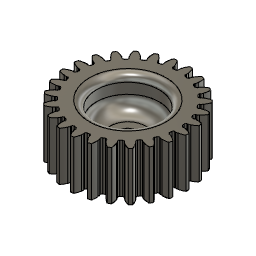
_motor gear.89c0d897-75a3-4985-b3bd-b82dc4103b69 (Autodesk Fusion 360 design; units mm, degrees)
description: Spur Gear; Module: 1.270000; Num Teeth: 25; Pressure Angle: 20.000000;
Autodesk Fusion 360 part; units mm, degrees
sketch "Sketch1" plane through (0, 0, 0) normal (0, 1, 0) x (1, 0, 0) in component "Spur Gear (25 teeth)"
  circle A0 centre (0, 0) radius 15.875 construction
sketch "sketch 16717" plane through (0, 0, 0) normal (0, 1, 0) x (1, 0, 0)
  arc A0 (14.1346, -2.0844) -> (14.4612, -2.5368) centre (14.5304, -2.1428) ccw
  spline S0 degree 3 poles (16.7153, -3.8203) (16.1288, -3.2859) (15.6262, -2.9744) (15.269, -2.7969) knots 0 0 0 0 1 1 1 1
  circle A1 centre (0, 0) radius 2.5
  line L0 (14.7175, -2.5817) -> (14.4612, -2.5368)
  arc A2 (14.1346, -2.0844) -> (14.2089, -1.4962) centre (0, 0) ccw
  spline S1 degree 3 poles (12.0329, -9.8069) (11.842, -9.5326) (11.7016, -9.3961) (11.6533, -9.3526) knots 0 0 0 0 1 1 1 1
  arc A3 (11.3821, -8.636) -> (11.4504, -9.1897) centre (11.7008, -8.8778) ccw
  arc A4 (11.3821, -8.636) -> (11.7306, -8.1563) centre (0, 0) ccw
  arc A5 (12.2783, -8.0502) -> (11.7306, -8.1563) centre (12.059, -8.3847) ccw
  arc A6 (14.8001, -8.6575) -> (15.2401, -7.8572) centre (0, 0) ccw
  spline S2 degree 3 poles (13.0445, -8.4135) (13.4271, -8.5286) (14.0067, -8.6456) (14.8001, -8.6575) knots 0 0 0 0 1 1 1 1
  spline S3 degree 3 poles (12.8073, -11.4004) (12.5507, -10.6496) (12.2604, -10.1345) (12.0329, -9.8069) knots 0 0 0 0 1 1 1 1
  spline S4 degree 3 poles (15.269, -2.7969) (14.9696, -2.6485) (14.7808, -2.5966) (14.7175, -2.5817) knots 0 0 0 0 1 1 1 1
  line L1 (11.6533, -9.3526) -> (11.4504, -9.1897)
  arc A7 (13.1722, -5.5341) -> (13.3761, -6.0534) centre (13.541, -5.689) ccw
  arc A8 (13.8946, -4.7438) -> (13.3904, -4.9828) centre (13.7653, -5.1223) ccw
  arc A9 (-4.1322, 13.6769) -> (-4.6961, 13.4937) centre (0, 0) ccw
  spline S5 degree 3 poles (-3.9705, 15.0067) (-3.9773, 14.6726) (-3.9439, 14.4796) (-3.9304, 14.416) knots 0 0 0 0 1 1 1 1
  arc A10 (-4.1322, 13.6769) -> (-3.862, 14.165) centre (-4.2479, 14.0598) ccw
  spline S6 degree 3 poles (14.727, -4.9052) (15.1263, -4.9214) (15.7167, -4.8906) (16.4882, -4.7049) knots 0 0 0 0 1 1 1 1
  line L2 (13.6131, -6.1607) -> (13.3761, -6.0534)
  spline S7 degree 3 poles (15.2401, -7.8572) (14.8049, -7.1938) (14.3955, -6.7671) (14.0937, -6.5063) knots 0 0 0 0 1 1 1 1
  spline S8 degree 3 poles (14.0937, -6.5063) (13.8406, -6.2881) (13.6707, -6.1908) (13.6131, -6.1607) knots 0 0 0 0 1 1 1 1
  arc A11 (13.1722, -5.5341) -> (13.3904, -4.9828) centre (0, 0) ccw
  spline S9 degree 3 poles (14.1408, -4.8278) (14.2034, -4.8453) (14.3939, -4.8907) (14.727, -4.9052) knots 0 0 0 0 1 1 1 1
  line L3 (12.2783, -8.0502) -> (12.4959, -8.1928)
  spline S10 degree 3 poles (12.4959, -8.1928) (12.5522, -8.2253) (12.7254, -8.3167) (13.0445, -8.4135) knots 0 0 0 0 1 1 1 1
  spline S11 degree 3 poles (-1.6525, 14.8505) (-1.6634, 14.9146) (-1.7034, 15.1064) (-1.8321, 15.4139) knots 0 0 0 0 1 1 1 1
  spline S12 degree 3 poles (-1.8321, 15.4139) (-1.9874, 15.7821) (-2.2667, 16.3033) (-2.7632, 16.9222) knots 0 0 0 0 1 1 1 1
  line L4 (13.8946, -4.7438) -> (14.1408, -4.8278)
  arc A12 (16.4882, -4.7049) -> (16.7153, -3.8203) centre (0, 0) ccw
  arc A13 (-2.7632, 16.9222) -> (-3.6603, 16.7511) centre (0, 0) ccw
  spline S13 degree 3 poles (-3.6603, 16.7511) (-3.8941, 15.9928) (-3.9619, 15.4055) (-3.9705, 15.0067) knots 0 0 0 0 1 1 1 1
  spline S14 degree 3 poles (-5.6078, 14.474) (-5.8498, 14.792) (-6.25, 15.2273) (-6.8848, 15.7034) knots 0 0 0 0 1 1 1 1
  spline S15 degree 3 poles (-7.5778, 13.5478) (-7.5012, 13.2225) (-7.4209, 13.0439) (-7.392, 12.9856) knots 0 0 0 0 1 1 1 1
  spline S16 degree 3 poles (-7.7111, 15.3145) (-7.749, 14.522) (-7.6687, 13.9362) (-7.5778, 13.5478) knots 0 0 0 0 1 1 1 1
  spline S17 degree 3 poles (-8.6024, 12.2175) (-8.6428, 12.2685) (-8.7702, 12.4172) (-9.0312, 12.6247) knots 0 0 0 0 1 1 1 1
  arc A14 (-7.4037, 12.2196) -> (-7.2633, 12.7596) centre (-7.611, 12.5617) ccw
  arc A15 (-7.4037, 12.2196) -> (-7.9043, 11.9019) centre (0, 0) ccw
  spline S18 degree 3 poles (-10.7089, 11.2377) (-10.5539, 10.9416) (-10.4317, 10.7886) (-10.3892, 10.7394) knots 0 0 0 0 1 1 1 1
  line L5 (-10.3892, 10.7394) -> (-10.2083, 10.5524)
  spline S19 degree 3 poles (-11.2774, 12.9157) (-11.117, 12.1386) (-10.8935, 11.5912) (-10.7089, 11.2377) knots 0 0 0 0 1 1 1 1
  spline S20 degree 3 poles (-9.0312, 12.6247) (-9.3447, 12.8725) (-9.8405, 13.1947) (-10.5738, 13.4978) knots 0 0 0 0 1 1 1 1
  arc A16 (-10.5738, 13.4978) -> (-11.2774, 12.9157) centre (0, 0) ccw
  arc A17 (-5.2016, 13.7298) -> (-4.6961, 13.4937) centre (-4.8275, 13.8715) ccw
  arc A18 (-6.8848, 15.7034) -> (-7.7111, 15.3145) centre (0, 0) ccw
  line L6 (-5.2016, 13.7298) -> (-5.2938, 13.973)
  line L7 (-7.392, 12.9856) -> (-7.2633, 12.7596)
  line L8 (-3.9304, 14.416) -> (-3.862, 14.165)
  arc A19 (-8.4526, 12.0048) -> (-7.9043, 11.9019) centre (-8.1256, 12.2351) ccw
  line L9 (-8.4526, 12.0048) -> (-8.6024, 12.2175)
  spline S21 degree 3 poles (-5.2938, 13.973) (-5.3202, 14.0324) (-5.4067, 14.2082) (-5.6078, 14.474) knots 0 0 0 0 1 1 1 1
  arc A20 (-12.3747, 7.1413) -> (-12.5119, 7.6822) centre (-12.7212, 7.3413) ccw
  spline S22 degree 3 poles (-13.9961, 6.7123) (-14.3902, 6.7785) (-14.9799, 6.8219) (-15.7685, 6.7343) knots 0 0 0 0 1 1 1 1
  spline S23 degree 3 poles (-11.3705, 9.6944) (-11.4223, 9.7337) (-11.5827, 9.846) (-11.8871, 9.9821) knots 0 0 0 0 1 1 1 1
  arc A21 (-10.21, 9.9945) -> (-10.6158, 9.5623) centre (0, 0) ccw
  spline S24 degree 3 poles (-17.0623, 1.6952) (-16.4134, 1.2386) (-15.8758, 0.9925) (-15.4992, 0.8612) knots 0 0 0 0 1 1 1 1
  arc A22 (-14.2844, 0.2964) -> (-14.2844, -0.2964) centre (0, 0) ccw
  spline S25 degree 3 poles (-13.1672, 8.2214) (-12.9434, 7.9732) (-12.7869, 7.8554) (-12.7336, 7.8183) knots 0 0 0 0 1 1 1 1
  line L10 (-14.925, 0.7168) -> (-14.6652, 0.7043)
  spline S26 degree 3 poles (-14.7981, 4.6886) (-14.5196, 4.5038) (-14.3388, 4.4286) (-14.2778, 4.4059) knots 0 0 0 0 1 1 1 1
  arc A23 (-11.1725, 9.5256) -> (-10.6158, 9.5623) centre (-10.913, 9.83) ccw
  spline S27 degree 3 poles (-16.1047, 5.8852) (-15.5897, 5.2815) (-15.1302, 4.9095) (-14.7981, 4.6886) knots 0 0 0 0 1 1 1 1
  spline S28 degree 3 poles (-15.2257, 3.0207) (-15.6238, 2.9868) (-16.2058, 2.8822) (-16.9478, 2.6013) knots 0 0 0 0 1 1 1 1
  spline S29 degree 3 poles (-15.4992, 0.8612) (-15.1835, 0.7515) (-14.9897, 0.7236) (-14.925, 0.7168) knots 0 0 0 0 1 1 1 1
  spline S30 degree 3 poles (-15.4985, -0.8607) (-15.8758, -0.9925) (-16.4134, -1.2386) (-17.0623, -1.6952) knots 0 0 0 0 1 1 1 1
  arc A24 (-13.5983, 10.4442) -> (-14.1351, 9.7054) centre (0, 0) ccw
  line L11 (-12.7336, 7.8183) -> (-12.5119, 7.6822)
  arc A25 (-17.0623, -1.6952) -> (-16.9478, -2.6013) centre (0, 0) ccw
  line L12 (-14.0293, -4.3292) -> (-14.2778, -4.4059)
  arc A26 (-16.9478, 2.6013) -> (-17.0623, 1.6952) centre (0, 0) ccw
  arc A27 (-13.9094, -3.2653) -> (-14.3796, -2.9649) centre (-14.2988, -3.3567) ccw
  spline S31 degree 3 poles (-11.8871, 9.9821) (-12.2524, 10.1442) (-12.8127, 10.3329) (-13.5983, 10.4442) knots 0 0 0 0 1 1 1 1
  line L13 (-14.2778, 4.4059) -> (-14.0293, 4.3292)
  spline S32 degree 3 poles (-16.9478, -2.6013) (-16.2058, -2.8822) (-15.6238, -2.9868) (-15.2264, -3.0204) knots 0 0 0 0 1 1 1 1
  line L14 (-14.6343, -3.0175) -> (-14.3796, -2.9649)
  arc A28 (-13.9094, -3.2653) -> (-13.7619, -3.8395) centre (0, 0) ccw
  spline S33 degree 3 poles (-14.6343, 3.0175) (-14.6987, 3.0269) (-14.8934, 3.0481) (-15.2257, 3.0207) knots 0 0 0 0 1 1 1 1
  spline S34 degree 3 poles (-15.2264, -3.0204) (-14.8934, -3.0481) (-14.6987, -3.0269) (-14.6343, -3.0175) knots 0 0 0 0 1 1 1 1
  arc A29 (-12.3747, 7.1413) -> (-12.6603, 6.6218) centre (0, 0) ccw
  line L15 (-11.1725, 9.5256) -> (-11.3705, 9.6944)
  arc A30 (-15.7685, 6.7343) -> (-16.1047, 5.8852) centre (0, 0) ccw
  spline S35 degree 3 poles (-13.4242, 6.5621) (-13.4841, 6.5872) (-13.6674, 6.6562) (-13.9961, 6.7123) knots 0 0 0 0 1 1 1 1
  line L16 (-13.1905, 6.4478) -> (-13.4242, 6.5621)
  arc A31 (-13.1905, 6.4478) -> (-12.6603, 6.6218) centre (-13.0148, 6.8072) ccw
  line L17 (-14.3796, 2.9649) -> (-14.6343, 3.0175)
  spline S36 degree 3 poles (-14.925, -0.7168) (-14.9897, -0.7236) (-15.1835, -0.7515) (-15.4985, -0.8607) knots 0 0 0 0 1 1 1 1
  arc A32 (-14.2844, 0.2964) -> (-14.6652, 0.7043) centre (-14.6843, 0.3047) ccw
  spline S37 degree 3 poles (-14.1351, 9.7054) (-13.7865, 8.9926) (-13.4339, 8.518) (-13.1672, 8.2214) knots 0 0 0 0 1 1 1 1
  line L18 (-14.6652, -0.7043) -> (-14.925, -0.7168)
  arc A33 (-13.7619, 3.8395) -> (-13.9094, 3.2653) centre (0, 0) ccw
  arc A34 (-14.3796, 2.9649) -> (-13.9094, 3.2653) centre (-14.2988, 3.3567) ccw
  arc A35 (-10.21, 9.9945) -> (-10.2083, 10.5524) centre (-10.4958, 10.2743) ccw
  arc A36 (-13.7619, 3.8395) -> (-14.0293, 4.3292) centre (-14.1472, 3.947) ccw
  arc A37 (-14.6652, -0.7043) -> (-14.2844, -0.2964) centre (-14.6843, -0.3047) ccw
  arc A38 (-4.6961, -13.4937) -> (-4.1322, -13.6769) centre (0, 0) ccw
  spline S38 degree 3 poles (2.0584, -15.386) (2.1069, -15.0554) (2.098, -14.8597) (2.0926, -14.7949) knots 0 0 0 0 1 1 1 1
  arc A39 (-12.6603, -6.6218) -> (-13.1905, -6.4478) centre (-13.0148, -6.8072) ccw
  arc A40 (3.4398, -14.2734) -> (2.9678, -13.9759) centre (3.0509, -14.3671) ccw
  arc A41 (-14.0293, -4.3292) -> (-13.7619, -3.8395) centre (-14.1472, -3.947) ccw
  arc A42 (-10.6158, -9.5623) -> (-11.1725, -9.5256) centre (-10.913, -9.83) ccw
  line L19 (-12.5119, -7.6822) -> (-12.7336, -7.8183)
  spline S39 degree 3 poles (-7.5778, -13.547) (-7.6687, -13.9362) (-7.749, -14.522) (-7.7111, -15.3145) knots 0 0 0 0 1 1 1 1
  arc A43 (-12.5119, -7.6822) -> (-12.3747, -7.1413) centre (-12.7212, -7.3413) ccw
  arc A44 (-0.2179, -14.6804) -> (-0.6011, -14.2749) centre (-0.6179, -14.6745) ccw
  arc A45 (-11.2774, -12.9157) -> (-10.5738, -13.4978) centre (0, 0) ccw
  line L20 (-5.2938, -13.973) -> (-5.2016, -13.7298)
  spline S40 degree 3 poles (-3.9708, -15.0059) (-3.9619, -15.4055) (-3.8941, -15.9928) (-3.6603, -16.7511) knots 0 0 0 0 1 1 1 1
  spline S41 degree 3 poles (-13.5983, -10.4442) (-12.8127, -10.3329) (-12.2524, -10.1442) (-11.8879, -9.9822) knots 0 0 0 0 1 1 1 1
  line L21 (-0.2179, -14.6804) -> (-0.2218, -14.9405)
  spline S42 degree 3 poles (-11.8879, -9.9822) (-11.5827, -9.846) (-11.4223, -9.7337) (-11.3705, -9.6944) knots 0 0 0 0 1 1 1 1
  spline S43 degree 3 poles (-0.1142, -15.522) (-0.0063, -15.9068) (0.2055, -16.4588) (0.6205, -17.1351) knots 0 0 0 0 1 1 1 1
  arc A46 (-12.6603, -6.6218) -> (-12.3747, -7.1413) centre (0, 0) ccw
  arc A47 (0.6205, -17.1351) -> (1.532, -17.0777) centre (0, 0) ccw
  arc A48 (-14.1351, -9.7054) -> (-13.5983, -10.4442) centre (0, 0) ccw
  arc A49 (-7.2633, -12.7596) -> (-7.4037, -12.2196) centre (-7.611, -12.5617) ccw
  arc A50 (-7.7111, -15.3145) -> (-6.8848, -15.7034) centre (0, 0) ccw
  spline S44 degree 3 poles (-6.8848, -15.7034) (-6.25, -15.2273) (-5.8498, -14.792) (-5.6085, -14.4745) knots 0 0 0 0 1 1 1 1
  spline S45 degree 3 poles (-15.7685, -6.7343) (-14.9799, -6.8219) (-14.3902, -6.7785) (-13.9969, -6.7121) knots 0 0 0 0 1 1 1 1
  arc A51 (-4.6961, -13.4937) -> (-5.2016, -13.7298) centre (-4.8275, -13.8715) ccw
  line L22 (-10.2083, -10.5524) -> (-10.3892, -10.7394)
  arc A52 (-16.1047, -5.8852) -> (-15.7685, -6.7343) centre (0, 0) ccw
  line L23 (-13.4242, -6.5621) -> (-13.1905, -6.4478)
  arc A53 (-1.1928, -14.2376) -> (-1.6237, -14.592) centre (-1.2262, -14.6362) ccw
  arc A54 (-10.2083, -10.5524) -> (-10.21, -9.9945) centre (-10.4958, -10.2743) ccw
  arc A55 (-10.6158, -9.5623) -> (-10.21, -9.9945) centre (0, 0) ccw
  spline S46 degree 3 poles (-14.7976, -4.688) (-15.1302, -4.9095) (-15.5897, -5.2815) (-16.1047, -5.8852) knots 0 0 0 0 1 1 1 1
  line L24 (-11.3705, -9.6944) -> (-11.1725, -9.5256)
  spline S47 degree 3 poles (-10.5738, -13.4978) (-9.8405, -13.1947) (-9.3447, -12.8725) (-9.032, -12.6249) knots 0 0 0 0 1 1 1 1
  line L25 (-7.2633, -12.7596) -> (-7.392, -12.9856)
  spline S48 degree 3 poles (-1.8327, -15.4145) (-1.7034, -15.1064) (-1.6634, -14.9146) (-1.6525, -14.8505) knots 0 0 0 0 1 1 1 1
  arc A56 (-1.1928, -14.2376) -> (-0.6011, -14.2749) centre (0, 0) ccw
  spline S49 degree 3 poles (-14.2778, -4.4059) (-14.3388, -4.4286) (-14.5196, -4.5038) (-14.7976, -4.688) knots 0 0 0 0 1 1 1 1
  line L26 (3.4398, -14.2734) -> (3.5007, -14.5263)
  arc A57 (-3.862, -14.165) -> (-4.1322, -13.6769) centre (-4.2479, -14.0598) ccw
  spline S50 degree 3 poles (-13.1668, -8.2207) (-13.4339, -8.518) (-13.7865, -8.9926) (-14.1351, -9.7054) knots 0 0 0 0 1 1 1 1
  arc A58 (-3.6603, -16.7511) -> (-2.7632, -16.9222) centre (0, 0) ccw
  spline S51 degree 3 poles (-3.9304, -14.416) (-3.9439, -14.4796) (-3.9773, -14.6726) (-3.9708, -15.0059) knots 0 0 0 0 1 1 1 1
  line L27 (-1.6525, -14.8505) -> (-1.6237, -14.592)
  arc A59 (-7.9043, -11.9019) -> (-8.4526, -12.0048) centre (-8.1256, -12.2351) ccw
  spline S52 degree 3 poles (-10.3892, -10.7394) (-10.4317, -10.7886) (-10.5539, -10.9416) (-10.7088, -11.2369) knots 0 0 0 0 1 1 1 1
  spline S53 degree 3 poles (-12.7336, -7.8183) (-12.7869, -7.8554) (-12.9434, -7.9732) (-13.1668, -8.2207) knots 0 0 0 0 1 1 1 1
  arc A60 (-7.9043, -11.9019) -> (-7.4037, -12.2196) centre (0, 0) ccw
  spline S54 degree 3 poles (-10.7088, -11.2369) (-10.8935, -11.5912) (-11.117, -12.1386) (-11.2774, -12.9157) knots 0 0 0 0 1 1 1 1
  line L28 (-3.862, -14.165) -> (-3.9304, -14.416)
  arc A61 (2.3854, -14.087) -> (2.9678, -13.9759) centre (0, 0) ccw
  line L29 (-8.6024, -12.2175) -> (-8.4526, -12.0048)
  spline S55 degree 3 poles (-0.2218, -14.9405) (-0.2191, -15.0055) (-0.2034, -15.2007) (-0.1142, -15.522) knots 0 0 0 0 1 1 1 1
  line L30 (2.0926, -14.7949) -> (2.0562, -14.5374)
  spline S56 degree 3 poles (1.532, -17.0777) (1.859, -16.3548) (1.9999, -15.7805) (2.0584, -15.386) knots 0 0 0 0 1 1 1 1
  arc A62 (4.8623, -16.4424) -> (5.7309, -16.1602) centre (0, 0) ccw
  spline S57 degree 3 poles (3.7496, -15.0627) (3.9498, -15.4086) (4.2922, -15.8906) (4.8623, -16.4424) knots 0 0 0 0 1 1 1 1
  spline S58 degree 3 poles (-13.9969, -6.7121) (-13.6674, -6.6562) (-13.4841, -6.5872) (-13.4242, -6.5621) knots 0 0 0 0 1 1 1 1
  spline S59 degree 3 poles (-7.392, -12.9856) (-7.4209, -13.0439) (-7.5012, -13.2225) (-7.5778, -13.547) knots 0 0 0 0 1 1 1 1
  spline S60 degree 3 poles (-2.7632, -16.9222) (-2.2667, -16.3033) (-1.9874, -15.7821) (-1.8327, -15.4145) knots 0 0 0 0 1 1 1 1
  arc A63 (2.3854, -14.087) -> (2.0562, -14.5374) centre (2.4522, -14.4813) ccw
  spline S61 degree 3 poles (-5.6085, -14.4745) (-5.4067, -14.2082) (-5.3202, -14.0324) (-5.2938, -13.973) knots 0 0 0 0 1 1 1 1
  spline S62 degree 3 poles (-9.032, -12.6249) (-8.7702, -12.4172) (-8.6428, -12.2685) (-8.6024, -12.2175) knots 0 0 0 0 1 1 1 1
  arc A64 (5.8138, -13.0512) -> (6.3502, -12.7987) centre (0, 0) ccw
  spline S63 degree 3 poles (5.7309, -16.1602) (5.8678, -15.3786) (5.8615, -14.7874) (5.82, -14.3907) knots 0 0 0 0 1 1 1 1
  line L31 (11.4504, 9.1897) -> (11.6533, 9.3526)
  arc A65 (11.7306, 8.1563) -> (12.2783, 8.0502) centre (12.059, 8.3847) ccw
  arc A66 (6.8814, -12.9696) -> (6.3502, -12.7987) centre (6.528, -13.157) ccw
  arc A67 (11.7306, 8.1563) -> (11.3821, 8.636) centre (0, 0) ccw
  spline S64 degree 3 poles (15.4842, -1.0886) (15.875, -1.0051) (16.4392, -0.8284) (17.1402, -0.4566) knots 0 0 0 0 1 1 1 1
  line L32 (13.3761, 6.0534) -> (13.6131, 6.1607)
  arc A68 (13.3904, 4.9828) -> (13.8946, 4.7438) centre (13.7653, 5.1223) ccw
  spline S65 degree 3 poles (14.7175, 2.5817) (14.7808, 2.5966) (14.9696, 2.6485) (15.2685, 2.7964) knots 0 0 0 0 1 1 1 1
  arc A69 (-0.6011, 14.2749) -> (-1.1928, 14.2376) centre (0, 0) ccw
  spline S66 degree 3 poles (12.0327, 9.8061) (12.2604, 10.1345) (12.5507, 10.6496) (12.8073, 11.4004) knots 0 0 0 0 1 1 1 1
  line L33 (5.7062, -13.8097) -> (5.6069, -13.5693)
  spline S67 degree 3 poles (9.5697, -14.2273) (9.508, -13.4362) (9.3548, -12.8651) (9.216, -12.4912) knots 0 0 0 0 1 1 1 1
  line L34 (-0.2218, 14.9405) -> (-0.2179, 14.6804)
  spline S68 degree 3 poles (14.0933, 6.5056) (14.3955, 6.7671) (14.8049, 7.1938) (15.2401, 7.8572) knots 0 0 0 0 1 1 1 1
  arc A70 (12.1821, -12.0662) -> (12.8073, -11.4004) centre (0, 0) ccw
  spline S69 degree 3 poles (5.82, -14.3907) (5.7849, -14.0584) (5.7276, -13.8711) (5.7062, -13.8097) knots 0 0 0 0 1 1 1 1
  arc A71 (12.8073, 11.4004) -> (12.1821, 12.0662) centre (0, 0) ccw
  arc A72 (16.7153, 3.8203) -> (16.4882, 4.7049) centre (0, 0) ccw
  arc A73 (-0.6011, 14.2749) -> (-0.2179, 14.6804) centre (-0.6179, 14.6745) ccw
  line L35 (14.6378, -1.1393) -> (14.8971, -1.1595)
  arc A74 (17.1402, -0.4566) -> (17.1402, 0.4566) centre (0, 0) ccw
  arc A75 (13.3904, 4.9828) -> (13.1722, 5.5341) centre (0, 0) ccw
  arc A76 (9.8906, -10.8508) -> (9.3336, -10.8174) centre (9.595, -11.1202) ccw
  arc A77 (5.8138, -13.0512) -> (5.6069, -13.5693) centre (5.9766, -13.4165) ccw
  arc A78 (14.2089, 1.4962) -> (14.6378, 1.1393) centre (14.6067, 1.5381) ccw
  spline S70 degree 3 poles (14.8971, -1.1595) (14.9621, -1.1608) (15.158, -1.1575) (15.4842, -1.0886) knots 0 0 0 0 1 1 1 1
  spline S71 degree 3 poles (-0.1137, 15.5227) (-0.2034, 15.2007) (-0.2191, 15.0055) (-0.2218, 14.9405) knots 0 0 0 0 1 1 1 1
  line L36 (14.8971, 1.1595) -> (14.6378, 1.1393)
  arc A79 (14.4612, 2.5368) -> (14.1346, 2.0844) centre (14.5304, 2.1428) ccw
  spline S72 degree 3 poles (3.5007, -14.5263) (3.5195, -14.5886) (3.5833, -14.7738) (3.7496, -15.0627) knots 0 0 0 0 1 1 1 1
  spline S73 degree 3 poles (7.0033, -13.1994) (7.037, -13.255) (7.1448, -13.4185) (7.3777, -13.657) knots 0 0 0 0 1 1 1 1
  line L37 (9.8906, -10.8508) -> (10.0658, -11.043)
  spline S74 degree 3 poles (0.6205, 17.1351) (0.2055, 16.4588) (-0.0063, 15.9068) (-0.1137, 15.5227) knots 0 0 0 0 1 1 1 1
  arc A80 (14.2089, 1.4962) -> (14.1346, 2.0844) centre (0, 0) ccw
  spline S75 degree 3 poles (16.4882, 4.7049) (15.7167, 4.8906) (15.1263, 4.9214) (14.7278, 4.9049) knots 0 0 0 0 1 1 1 1
  spline S76 degree 3 poles (10.0658, -11.043) (10.1123, -11.0885) (10.2574, -11.2201) (10.5423, -11.3932) knots 0 0 0 0 1 1 1 1
  arc A81 (8.8768, -11.1953) -> (8.8053, -11.7486) centre (9.1253, -11.5087) ccw
  spline S77 degree 3 poles (14.7278, 4.9049) (14.3939, 4.8907) (14.2034, 4.8453) (14.1408, 4.8278) knots 0 0 0 0 1 1 1 1
  spline S78 degree 3 poles (10.5423, -11.3932) (10.8843, -11.5998) (11.4166, -11.8573) (12.1821, -12.0662) knots 0 0 0 0 1 1 1 1
  line L38 (14.4612, 2.5368) -> (14.7175, 2.5817)
  spline S79 degree 3 poles (13.6131, 6.1607) (13.6707, 6.1908) (13.8406, 6.2881) (14.0933, 6.5056) knots 0 0 0 0 1 1 1 1
  spline S80 degree 3 poles (13.0453, 8.4135) (12.7254, 8.3167) (12.5522, 8.2253) (12.4959, 8.1928) knots 0 0 0 0 1 1 1 1
  line L39 (-1.6237, 14.592) -> (-1.6525, 14.8505)
  arc A82 (14.6378, -1.1393) -> (14.2089, -1.4962) centre (14.6067, -1.5381) ccw
  line L40 (6.8814, -12.9696) -> (7.0033, -13.1994)
  spline S81 degree 3 poles (7.3777, -13.657) (7.6576, -13.9422) (8.1092, -14.3239) (8.7987, -14.7167) knots 0 0 0 0 1 1 1 1
  arc A83 (8.8768, -11.1953) -> (9.3336, -10.8174) centre (0, 0) ccw
  line L41 (8.9613, -11.9568) -> (8.8053, -11.7486)
  arc A84 (8.7987, -14.7167) -> (9.5697, -14.2273) centre (0, 0) ccw
  arc A85 (13.3761, 6.0534) -> (13.1722, 5.5341) centre (13.541, 5.689) ccw
  line L42 (14.1408, 4.8278) -> (13.8946, 4.7438)
  arc A86 (-1.6237, 14.592) -> (-1.1928, 14.2376) centre (-1.2262, 14.6362) ccw
  spline S82 degree 3 poles (15.4849, 1.0882) (15.158, 1.1575) (14.9621, 1.1608) (14.8971, 1.1595) knots 0 0 0 0 1 1 1 1
  arc A87 (15.2401, 7.8572) -> (14.8001, 8.6575) centre (0, 0) ccw
  spline S83 degree 3 poles (17.1402, 0.4566) (16.4392, 0.8284) (15.875, 1.0051) (15.4849, 1.0882) knots 0 0 0 0 1 1 1 1
  spline S84 degree 3 poles (9.216, -12.4912) (9.0993, -12.1781) (8.9972, -12.011) (8.9613, -11.9568) knots 0 0 0 0 1 1 1 1
  spline S85 degree 3 poles (15.2685, 2.7964) (15.6262, 2.9744) (16.1288, 3.2859) (16.7153, 3.8203) knots 0 0 0 0 1 1 1 1
  line L43 (12.4959, 8.1928) -> (12.2783, 8.0502)
  spline S86 degree 3 poles (14.8001, 8.6575) (14.0067, 8.6456) (13.4271, 8.5286) (13.0453, 8.4135) knots 0 0 0 0 1 1 1 1
  arc A88 (11.4504, 9.1897) -> (11.3821, 8.636) centre (11.7008, 8.8778) ccw
  arc A89 (2.9678, 13.9759) -> (2.3854, 14.087) centre (0, 0) ccw
  spline S87 degree 3 poles (11.6533, 9.3526) (11.7016, 9.3961) (11.842, 9.5326) (12.0327, 9.8061) knots 0 0 0 0 1 1 1 1
  spline S88 degree 3 poles (3.7502, 15.0633) (3.5833, 14.7738) (3.5195, 14.5886) (3.5007, 14.5263) knots 0 0 0 0 1 1 1 1
  spline S89 degree 3 poles (8.9613, 11.9568) (8.9972, 12.011) (9.0993, 12.1781) (9.216, 12.4904) knots 0 0 0 0 1 1 1 1
  arc A90 (5.6069, 13.5693) -> (5.8138, 13.0512) centre (5.9766, 13.4165) ccw
  line L44 (5.6069, 13.5693) -> (5.7062, 13.8097)
  spline S90 degree 3 poles (9.216, 12.4904) (9.3548, 12.8651) (9.508, 13.4362) (9.5697, 14.2273) knots 0 0 0 0 1 1 1 1
  line L45 (8.8053, 11.7486) -> (8.9613, 11.9568)
  arc A91 (9.3336, 10.8174) -> (9.8906, 10.8508) centre (9.595, 11.1202) ccw
  spline S91 degree 3 poles (10.5431, 11.3934) (10.2574, 11.2201) (10.1123, 11.0885) (10.0658, 11.043) knots 0 0 0 0 1 1 1 1
  spline S92 degree 3 poles (7.3784, 13.6574) (7.1448, 13.4185) (7.037, 13.255) (7.0033, 13.1994) knots 0 0 0 0 1 1 1 1
  spline S93 degree 3 poles (2.0926, 14.7949) (2.098, 14.8597) (2.1069, 15.0554) (2.0587, 15.3853) knots 0 0 0 0 1 1 1 1
  line L46 (3.5007, 14.5263) -> (3.4398, 14.2734)
  arc A92 (9.5697, 14.2273) -> (8.7987, 14.7167) centre (0, 0) ccw
  line L47 (10.0658, 11.043) -> (9.8906, 10.8508)
  spline S94 degree 3 poles (2.0587, 15.3853) (1.9999, 15.7805) (1.859, 16.3548) (1.532, 17.0777) knots 0 0 0 0 1 1 1 1
  spline S95 degree 3 poles (5.8202, 14.3899) (5.8615, 14.7874) (5.8678, 15.3786) (5.7309, 16.1602) knots 0 0 0 0 1 1 1 1
  spline S96 degree 3 poles (8.7987, 14.7167) (8.1092, 14.3239) (7.6576, 13.9422) (7.3784, 13.6574) knots 0 0 0 0 1 1 1 1
  line L48 (7.0033, 13.1994) -> (6.8814, 12.9696)
  arc A93 (6.3502, 12.7987) -> (5.8138, 13.0512) centre (0, 0) ccw
  arc A94 (8.8053, 11.7486) -> (8.8768, 11.1953) centre (9.1253, 11.5087) ccw
  arc A95 (5.7309, 16.1602) -> (4.8623, 16.4424) centre (0, 0) ccw
  spline S97 degree 3 poles (12.1821, 12.0662) (11.4166, 11.8573) (10.8843, 11.5998) (10.5431, 11.3934) knots 0 0 0 0 1 1 1 1
  arc A96 (1.532, 17.0777) -> (0.6205, 17.1351) centre (0, 0) ccw
  arc A97 (9.3336, 10.8174) -> (8.8768, 11.1953) centre (0, 0) ccw
  arc A98 (6.3502, 12.7987) -> (6.8814, 12.9696) centre (6.528, 13.157) ccw
  spline S98 degree 3 poles (4.8623, 16.4424) (4.2922, 15.8906) (3.9498, 15.4086) (3.7502, 15.0633) knots 0 0 0 0 1 1 1 1
  line L49 (2.0562, 14.5374) -> (2.0926, 14.7949)
  spline S99 degree 3 poles (5.7062, 13.8097) (5.7276, 13.8711) (5.7849, 14.0584) (5.8202, 14.3899) knots 0 0 0 0 1 1 1 1
  arc A99 (2.0562, 14.5374) -> (2.3854, 14.087) centre (2.4522, 14.4813) ccw
  arc A100 (2.9678, 13.9759) -> (3.4398, 14.2734) centre (3.0509, 14.3671) ccw
  circle A101 centre (0, 0) radius 9
  circle A102 centre (0, 0) radius 8.5
  circle A103 centre (0, 0) radius 2.6
  constraint concentric A87 A101
  constraint concentric A74 A102
extrude "Extrude5" add sketch "sketch 16717" along normal blind 14 contours A0 S0 L0 A2 S1 A3 A4 A5 A6 S2 S3 S4 L1 A7 A8 A9 S5 A10 S6 L2 S7 S8 A11 S9 L3 S10 S11 S12 L4 A12 A13 S13 S14 S15 S16 S17 A14 A15 S18 L5 S19 S20 A16 A17 A18 L6 L7 L8 A19 L9 S21 A20 S22 S23 A21 S24 A22 S25 L10 S26 A23 S27 S28 S29 S30 A24 L11 A25 L12 A26 A27 S31 L13 S32 L14 A28 S33 S34 A29 L15 A30 S35 L16 A31 L17 S36 A32 S37 L18 A33 A34 A35 A36 A37 A38 S38 A39 A40 A41 A42 L19 S39 A43 A44 A45 L20 S40 S41 L21 S42 S43 A46 A47 A48 A49 A50 S44 S45 A51 L22 A52 L23 A53 A54 A55 S46 L24 S47 L25 S48 A56 S49 L26 A57 S50 A58 S51 L27 A59 S52 S53 A60 S54 L28 A61 L29 S55 L30 S56 A62 S57 S58 S59 S60 A63 S61 S62 A64 S63 L31 A65 A66 A67 S64 L32 A68 S65 A69 S66 L33 S67 L34 S68 A70 S69 A71 A72 A73 L35 A74 A75 A76 A77 A78 S70 S71 L36 A79 S72 S73 L37 S74 A80 S75 S76 A81 S77 S78 L38 S79 S80 L39 A82 L40 S81 A83 L41 A84 A85 L42 A86 S82 A87 S83 S84 S85 L43 S86 A88 A89 S87 S88 S89 A90 L44 S90 L45 A91 S91 S92 S93 L46 A92 L47 S94 S95 S96 L48 A93 A94 A95 S97 A96 A97 A98 S98 L49 S99 A99 A100 | A101 | A102 in component "Spur Gear (25 teeth)"
extrude "Extrude6" cut sketch "sketch 16717" along normal blind 11 from surface at 5 contours A101 | A102 in component "Spur Gear (25 teeth)"
fillet "Fillet1" radius 4 1 edges at (-8.3909, 5, 3.2545) in component "Spur Gear (25 teeth)"
fillet "Fillet2" radius 2 1 edges at (-8.3909, 14, -3.2545) in component "Spur Gear (25 teeth)"
hole "Hole1" at (0, 0, 0) direction (0, 1, 0) diameter 5.4 depth 20 tip angle 118 in component "Spur Gear (25 teeth)"
extrude "Extrude8" [suppressed]
extrude "Extrude9" [suppressed]
chamfer "Chamfer1" [suppressed]
extrude "Extrude10" [suppressed]
extrude "Extrude11" [suppressed]
extrude "Extrude12" [suppressed]
extrude "Extrude13" [suppressed]
extrude "Extrude14" [suppressed]
extrude "Extrude15" [suppressed]
extrude "Extrude16" [suppressed]
extrude "Extrude17" [suppressed]
extrude "Extrude18" [suppressed]
combine "Combine1" [suppressed]
component "Spur Gear (25 teeth)" placed x (1, 0, 0) y (0, 1, 0) z (0, 0, 1) at (0, 0, 0)
